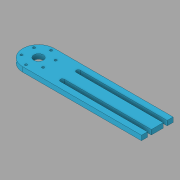
# Autodesk Inventor part: work-area--holder--motor
Saved by Autodesk Inventor 2019 (Build 230136000, 136)
## iProperties
Created: 2023-08-22
Part Number: work-area--holder--motor
Material: Generic
Document SubType Name: Modeling
Designer: m00
Density: 1 g/cm^3
Appearance: Default
Author: m00
Autodesk Inventor part; units mm, degrees
ref_plane "YZ Plane" through (0, 0, 0) normal (1, 0, 0) x (0, 1, 0)
ref_plane "XZ Plane" through (0, 0, 0) normal (0, 1, 0) x (-1, 0, 0)
ref_plane "XY Plane" through (0, 0, 0) normal (0, 0, 1) x (1, 0, 0)
sketch "sketch1--base" plane through (0, 0, 0) normal (0, 1, 0) x (-1, 0, 0)
  line L0 (-18.2322, -18.2322) -> (18.2322, 18.2322) construction
  line L1 (21.7082, -21.7082) -> (-21.7082, 21.7082) construction
  line L2 (-20, -20) -> (20, -20) construction
  line L3 (20, -20) -> (20, 20) construction
  line L4 (20, 20) -> (-20, 20) construction
  line L5 (-20, 20) -> (-20, -20) construction
  line L6 (-20, -20) -> (20, 20) construction
  line L7 (20, -20) -> (-20, 20) construction
  line L8 (-21.7678, -21.7678) -> (21.7678, 21.7678) construction
  line L9 (21.7678, -21.7678) -> (-21.7678, 21.7678) construction
  circle A0 centre (-20, 20) radius 2.5 construction
  circle A1 centre (20, 20) radius 2.5 construction
  circle A2 centre (20, -20) radius 2.5 construction
  circle A3 centre (-20, -20) radius 2.5 construction
  arc A4 (17.5, 20) -> (20, 17.5) centre (20, 20) ccw
  arc A5 (20, -17.5) -> (17.5, -20) centre (20, -20) ccw
  arc A6 (-20, 17.5) -> (-17.5, 20) centre (-20, 20) ccw
  arc A7 (-17.5, -20) -> (-20, -17.5) centre (-20, -20) ccw
  line L10 (-17.5, -20) -> (17.5, -20)
  line L11 (-20, -17.5) -> (-20, 17.5)
  line L12 (0, -20) -> (0, 20) construction
  line L13 (20, 0) -> (-20, 0) construction
  line L14 (20, -17.5) -> (20, 17.5)
  line L15 (17.5, 20) -> (-17.5, 20)
  point P0 (0, 0)
  point P1 (20, 0)
  dimension "d6" = 40
  dimension "screw__diameter" = 5
  dimension "d24" = 40
  constraints: 32 end point, 22 point on circle, 12 midpoint, 8 centre point, 7 equal radius, 7 point on line, 4 collinear, 3 coincident, 2 horizontal, 2 parallel, 1 concentric, 1 perpendicular, 1 vertical
  measures "d6" distance of L2.start L2.end
  measures "screw__diameter" diameter of A1
  measures "d24" distance between parallel lines of L15 L10
sketch "sketch2--component" plane through (0, 0, 0) normal (0, 1, 0) x (-1, 0, 0)
  circle A0 centre (0, 0) radius 18.5
  circle A1 centre (0, 0) radius 15.8 construction
  circle A2 centre (0, -15.8) radius 1.5
  circle A3 centre (0, 0) radius 17.3 construction
  circle A4 centre (13.6832, -7.9) radius 1.5
  circle A5 centre (13.6832, 7.9) radius 1.5
  circle A6 centre (0, 15.8) radius 1.5
  circle A7 centre (-13.6832, 7.9) radius 1.5
  circle A8 centre (-13.6832, -7.9) radius 1.5
  circle A9 centre (0, 0) radius 6
  dimension "d40" = 37
  dimension "d41" = 1.2
  dimension "d42" = 3
  dimension "d45" = 360
  dimension "d49" = 12
  constraints: 9 centre point, 6 coincident, 2 vertical alignment, 1 tangent, 15 other
  measures "d40" diameter of A0
  measures "d41" radial gap between concentric circles of A0 A3
  measures "d42" diameter of A2
  measures "d49" diameter of A9
sketch "Sketch3--union" plane through (0, 0, 0) normal (0, 1, 0) x (-1, 0, 0)
  circle A0 centre (13.6832, 7.9) radius 1.5 projected
  circle A1 centre (13.6832, -7.9) radius 1.5 projected
  circle A2 centre (0, -15.8) radius 1.5 projected
  circle A3 centre (-13.6832, -7.9) radius 1.5 projected
  circle A4 centre (-13.6832, 7.9) radius 1.5 projected
  circle A5 centre (0, 15.8) radius 1.5 projected
  circle A6 centre (0, 0) radius 20 construction
  line L0 (20, -20) -> (20, 20) construction
  arc A7 (0, -20) -> (0, 20) centre (0, 0) ccw
  line L1 (0, -20) -> (0, 20) construction
  line L2 (0, 20) -> (-150, 20)
  line L3 (-150, -20) -> (0, -20)
  line L4 (-20, 20) -> (-20, -20) construction
  line L5 (-20, 20) -> (-150, 0) construction
  line L6 (-20, 0) -> (-150, 20) construction
  line L7 (20, 0) -> (-20, 0) construction
  circle A8 centre (20, 20) radius 2.5 construction
  circle A9 centre (0, 0) radius 6 projected
  line L8 (-132.5, 10) -> (-37.5, 10) construction
  line L9 (-132.5, 10) -> (-37.5, 10) construction
  line L10 (-150, 7.5) -> (-40, 7.5)
  line L11 (-40, 12.5) -> (-150, 12.5)
  arc A10 (-40, 7.5) -> (-40, 12.5) centre (-40, 10) ccw
  line L12 (-150, 20) -> (-150, 12.5)
  line L13 (-150, 7.5) -> (-150, 0)
  line L14 (-150, -7.5) -> (-40, -7.5)
  line L15 (-40, -12.5) -> (-150, -12.5)
  arc A11 (-40, -12.5) -> (-40, -7.5) centre (-40, -10) ccw
  line L16 (-150, -20) -> (-150, -12.5)
  line L17 (-150, -7.5) -> (-150, 0)
  point P0 (-85, 10)
  point P1 (-85, 10)
  point P2 (-85, 10)
  dimension "d52" = 2.5
  dimension "d53" = 130
  dimension "d54" = 20
  constraints: 30 end point, 7 point on circle, 6 midpoint, 5 symmetric about line, 4 centre point, 4 tangent, 3 horizontal, 2 collinear, 2 parallel, 2 perpendicular, 1 coincident, 1 point on line, 1 vertical, 1 other
  measures "d52" radius of A10
  measures "d53" distance between parallel lines of L4 L12
  measures "d54" distance from line of L4 A10.centre
extrude "Extrusion3--base" add sketch "Sketch3--union" along normal blind 6
equation "\"d6\" = module__size"
equation "\"d24\" = d6"
equation "\"d50\" = module__height"
equation "\"module__height\" = 6"
equation "\"module__size\" = 40"
body "Solid4"
